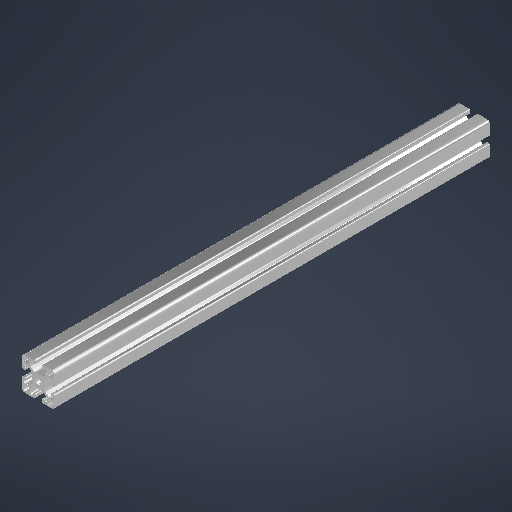
# Autodesk Inventor part: profileAluAvant2
Saved by Autodesk Inventor 2026.2 (Build 302298010, 298A)
## iProperties
Part Number: profileAluAvant2
Material: Générique
Document SubType Name: Modélisation
Designer: quent
Appearance: Par défaut
Author: quent
Autodesk Inventor part; units mm, degrees
ref_plane "Plan YZ" through (0, 0, 0) normal (1, 0, 0) x (0, 1, 0)
ref_plane "Plan XZ" through (0, 0, 0) normal (0, 1, 0) x (-1, 0, 0)
ref_plane "Plan XY" through (0, 0, 0) normal (0, 0, 1) x (1, 0, 0)
sketch "Esquisse1" plane through (0, 0, 0) normal (0, 0, 1) x (1, 0, 0)
  arc A0 (-0.1097, 10.4512) -> (1.0153, 9.3262) centre (1.0153, 10.4512) ccw
  line L0 (2.5153, 9.3262) -> (1.0153, 9.3262)
  arc A1 (2.5153, 9.3262) -> (3.2653, 10.0762) centre (2.5153, 10.0762) ccw
  line L1 (3.2653, 11.2012) -> (3.2653, 10.0762)
  arc A2 (3.2653, 11.2012) -> (2.8903, 11.5762) centre (2.8903, 11.2012) ccw
  line L2 (1.7653, 11.5762) -> (2.8903, 11.5762)
  arc A3 (1.3903, 11.9512) -> (1.7653, 11.5762) centre (1.7653, 11.9512) ccw
  arc A4 (3.2653, 13.8262) -> (1.3903, 11.9512) centre (3.2653, 11.9512) ccw
  line L3 (4.246, 13.8262) -> (3.2653, 13.8262)
  arc A5 (6.8976, 12.7279) -> (4.246, 13.8262) centre (4.246, 10.0762) ccw
  line L4 (7.9794, 11.6461) -> (6.8976, 12.7279)
  arc A6 (9.0778, 8.9944) -> (7.9794, 11.6461) centre (5.3278, 8.9944) ccw
  line L5 (9.0778, 3.658) -> (9.0778, 8.9944)
  arc A7 (7.9794, 1.0064) -> (9.0778, 3.658) centre (5.3278, 3.658) ccw
  line L6 (6.8976, -0.0754) -> (7.9794, 1.0064)
  arc A8 (4.246, -1.1738) -> (6.8976, -0.0754) centre (4.246, 2.5762) ccw
  line L7 (3.2653, -1.1738) -> (4.246, -1.1738)
  arc A9 (1.3903, 0.7012) -> (3.2653, -1.1738) centre (3.2653, 0.7012) ccw
  arc A10 (1.7653, 1.0762) -> (1.3903, 0.7012) centre (1.7653, 0.7012) ccw
  line L8 (2.8903, 1.0762) -> (1.7653, 1.0762)
  arc A11 (2.8903, 1.0762) -> (3.2653, 1.4512) centre (2.8903, 1.4512) ccw
  line L9 (3.2653, 2.5762) -> (3.2653, 1.4512)
  arc A12 (3.2653, 2.5762) -> (2.5153, 3.3262) centre (2.5153, 2.5762) ccw
  line L10 (1.0153, 3.3262) -> (2.5153, 3.3262)
  arc A13 (1.0153, 3.3262) -> (-0.1097, 2.2012) centre (1.0153, 2.2012) ccw
  line L11 (-0.1097, -5.6738) -> (-0.1097, 2.2012)
  arc A14 (-0.1097, -5.6738) -> (2.8903, -8.6738) centre (2.8903, -5.6738) ccw
  line L12 (10.7653, -8.6738) -> (2.8903, -8.6738)
  arc A15 (10.7653, -8.6738) -> (11.8903, -7.5488) centre (10.7653, -7.5488) ccw
  line L13 (11.8903, -6.0488) -> (11.8903, -7.5488)
  arc A16 (11.8903, -6.0488) -> (11.1403, -5.2988) centre (11.1403, -6.0488) ccw
  line L14 (10.0153, -5.2988) -> (11.1403, -5.2988)
  arc A17 (10.0153, -5.2988) -> (9.6403, -5.6738) centre (10.0153, -5.6738) ccw
  line L15 (9.6403, -6.7988) -> (9.6403, -5.6738)
  arc A18 (9.2653, -7.1738) -> (9.6403, -6.7988) centre (9.2653, -6.7988) ccw
  arc A19 (7.3903, -5.2988) -> (9.2653, -7.1738) centre (9.2653, -5.2988) ccw
  line L16 (7.3903, -4.3181) -> (7.3903, -5.2988)
  arc A20 (8.4886, -1.6664) -> (7.3903, -4.3181) centre (11.1403, -4.3181) ccw
  line L17 (9.5704, -0.5846) -> (8.4886, -1.6664)
  arc A21 (12.2221, 0.5137) -> (9.5704, -0.5846) centre (12.2221, -3.2363) ccw
  line L18 (17.5585, 0.5137) -> (12.2221, 0.5137)
  arc A22 (20.2101, -0.5846) -> (17.5585, 0.5137) centre (17.5585, -3.2363) ccw
  line L19 (21.2919, -1.6664) -> (20.2101, -0.5846)
  arc A23 (22.3903, -4.3181) -> (21.2919, -1.6664) centre (18.6403, -4.3181) ccw
  line L20 (22.3903, -5.2988) -> (22.3903, -4.3181)
  arc A24 (20.5153, -7.1738) -> (22.3903, -5.2988) centre (20.5153, -5.2988) ccw
  arc A25 (20.1403, -6.7988) -> (20.5153, -7.1738) centre (20.5153, -6.7988) ccw
  line L21 (20.1403, -5.6738) -> (20.1403, -6.7988)
  arc A26 (20.1403, -5.6738) -> (19.7653, -5.2988) centre (19.7653, -5.6738) ccw
  line L22 (18.6403, -5.2988) -> (19.7653, -5.2988)
  arc A27 (18.6403, -5.2988) -> (17.8903, -6.0488) centre (18.6403, -6.0488) ccw
  line L23 (17.8903, -7.5488) -> (17.8903, -6.0488)
  arc A28 (17.8903, -7.5488) -> (19.0153, -8.6738) centre (19.0153, -7.5488) ccw
  line L24 (26.8903, -8.6738) -> (19.0153, -8.6738)
  arc A29 (26.8903, -8.6738) -> (29.8903, -5.6738) centre (26.8903, -5.6738) ccw
  line L25 (29.8903, 2.2012) -> (29.8903, -5.6738)
  arc A30 (29.8903, 2.2012) -> (28.7653, 3.3262) centre (28.7653, 2.2012) ccw
  line L26 (27.2653, 3.3262) -> (28.7653, 3.3262)
  arc A31 (27.2653, 3.3262) -> (26.5153, 2.5762) centre (27.2653, 2.5762) ccw
  line L27 (26.5153, 1.4512) -> (26.5153, 2.5762)
  arc A32 (26.5153, 1.4512) -> (26.8903, 1.0762) centre (26.8903, 1.4512) ccw
  line L28 (28.0153, 1.0762) -> (26.8903, 1.0762)
  arc A33 (28.3903, 0.7012) -> (28.0153, 1.0762) centre (28.0153, 0.7012) ccw
  arc A34 (26.5153, -1.1738) -> (28.3903, 0.7012) centre (26.5153, 0.7012) ccw
  line L29 (25.5346, -1.1738) -> (26.5153, -1.1738)
  arc A35 (22.8829, -0.0754) -> (25.5346, -1.1738) centre (25.5346, 2.5762) ccw
  line L30 (21.8011, 1.0064) -> (22.8829, -0.0754)
  arc A36 (20.7028, 3.658) -> (21.8011, 1.0064) centre (24.4528, 3.658) ccw
  line L31 (20.7028, 8.9944) -> (20.7028, 3.658)
  arc A37 (21.8011, 11.6461) -> (20.7028, 8.9944) centre (24.4528, 8.9944) ccw
  line L32 (22.8829, 12.7279) -> (21.8011, 11.6461)
  arc A38 (25.5346, 13.8262) -> (22.8829, 12.7279) centre (25.5346, 10.0762) ccw
  line L33 (26.5153, 13.8262) -> (25.5346, 13.8262)
  arc A39 (28.3903, 11.9512) -> (26.5153, 13.8262) centre (26.5153, 11.9512) ccw
  arc A40 (28.0153, 11.5762) -> (28.3903, 11.9512) centre (28.0153, 11.9512) ccw
  line L34 (26.8903, 11.5762) -> (28.0153, 11.5762)
  arc A41 (26.8903, 11.5762) -> (26.5153, 11.2012) centre (26.8903, 11.2012) ccw
  line L35 (26.5153, 10.0762) -> (26.5153, 11.2012)
  arc A42 (26.5153, 10.0762) -> (27.2653, 9.3262) centre (27.2653, 10.0762) ccw
  line L36 (28.7653, 9.3262) -> (27.2653, 9.3262)
  arc A43 (28.7653, 9.3262) -> (29.8903, 10.4512) centre (28.7653, 10.4512) ccw
  line L37 (29.8903, 18.3262) -> (29.8903, 10.4512)
  arc A44 (29.8903, 18.3262) -> (26.8903, 21.3262) centre (26.8903, 18.3262) ccw
  line L38 (19.0153, 21.3262) -> (26.8903, 21.3262)
  arc A45 (19.0153, 21.3262) -> (17.8903, 20.2012) centre (19.0153, 20.2012) ccw
  line L39 (17.8903, 18.7012) -> (17.8903, 20.2012)
  arc A46 (17.8903, 18.7012) -> (18.6403, 17.9512) centre (18.6403, 18.7012) ccw
  line L40 (19.7653, 17.9512) -> (18.6403, 17.9512)
  arc A47 (19.7653, 17.9512) -> (20.1403, 18.3262) centre (19.7653, 18.3262) ccw
  line L41 (20.1403, 19.4512) -> (20.1403, 18.3262)
  arc A48 (20.5153, 19.8262) -> (20.1403, 19.4512) centre (20.5153, 19.4512) ccw
  arc A49 (22.3903, 17.9512) -> (20.5153, 19.8262) centre (20.5153, 17.9512) ccw
  line L42 (22.3903, 16.9705) -> (22.3903, 17.9512)
  arc A50 (21.2919, 14.3189) -> (22.3903, 16.9705) centre (18.6403, 16.9705) ccw
  line L43 (20.2101, 13.2371) -> (21.2919, 14.3189)
  arc A51 (17.5585, 12.1387) -> (20.2101, 13.2371) centre (17.5585, 15.8887) ccw
  line L44 (12.2221, 12.1387) -> (17.5585, 12.1387)
  arc A52 (9.5704, 13.2371) -> (12.2221, 12.1387) centre (12.2221, 15.8887) ccw
  line L45 (8.4886, 14.3189) -> (9.5704, 13.2371)
  arc A53 (7.3903, 16.9705) -> (8.4886, 14.3189) centre (11.1403, 16.9705) ccw
  line L46 (7.3903, 17.9512) -> (7.3903, 16.9705)
  arc A54 (9.2653, 19.8262) -> (7.3903, 17.9512) centre (9.2653, 17.9512) ccw
  arc A55 (9.6403, 19.4512) -> (9.2653, 19.8262) centre (9.2653, 19.4512) ccw
  line L47 (9.6403, 18.3262) -> (9.6403, 19.4512)
  arc A56 (9.6403, 18.3262) -> (10.0153, 17.9512) centre (10.0153, 18.3262) ccw
  line L48 (11.1403, 17.9512) -> (10.0153, 17.9512)
  arc A57 (11.1403, 17.9512) -> (11.8903, 18.7012) centre (11.1403, 18.7012) ccw
  line L49 (11.8903, 20.2012) -> (11.8903, 18.7012)
  arc A58 (11.8903, 20.2012) -> (10.7653, 21.3262) centre (10.7653, 20.2012) ccw
  line L50 (2.8903, 21.3262) -> (10.7653, 21.3262)
  arc A59 (2.8903, 21.3262) -> (-0.1097, 18.3262) centre (2.8903, 18.3262) ccw
  line L51 (-0.1097, 10.4512) -> (-0.1097, 18.3262)
  line L52 (23.7403, -6.9488) -> (23.7403, -2.8988)
  arc A60 (24.1153, -2.5238) -> (23.7403, -2.8988) centre (24.1153, -2.8988) ccw
  line L53 (24.1153, -2.5238) -> (28.1653, -2.5238)
  arc A61 (28.5403, -2.8988) -> (28.1653, -2.5238) centre (28.1653, -2.8988) ccw
  line L54 (28.5403, -2.8988) -> (28.5403, -5.6738)
  arc A62 (26.8903, -7.3238) -> (28.5403, -5.6738) centre (26.8903, -5.6738) ccw
  line L55 (26.8903, -7.3238) -> (24.1153, -7.3238)
  arc A63 (23.7403, -6.9488) -> (24.1153, -7.3238) centre (24.1153, -6.9488) ccw
  line L56 (1.6153, -2.5238) -> (5.6653, -2.5238)
  arc A64 (6.0403, -2.8988) -> (5.6653, -2.5238) centre (5.6653, -2.8988) ccw
  line L57 (6.0403, -2.8988) -> (6.0403, -6.9488)
  arc A65 (5.6653, -7.3238) -> (6.0403, -6.9488) centre (5.6653, -6.9488) ccw
  line L58 (5.6653, -7.3238) -> (2.8903, -7.3238)
  arc A66 (1.2403, -5.6738) -> (2.8903, -7.3238) centre (2.8903, -5.6738) ccw
  line L59 (1.2403, -5.6738) -> (1.2403, -2.8988)
  arc A67 (1.6153, -2.5238) -> (1.2403, -2.8988) centre (1.6153, -2.8988) ccw
  line L60 (6.0403, 19.6012) -> (6.0403, 15.5512)
  arc A68 (5.6653, 15.1762) -> (6.0403, 15.5512) centre (5.6653, 15.5512) ccw
  line L61 (5.6653, 15.1762) -> (1.6153, 15.1762)
  arc A69 (1.2403, 15.5512) -> (1.6153, 15.1762) centre (1.6153, 15.5512) ccw
  line L62 (1.2403, 15.5512) -> (1.2403, 18.3262)
  arc A70 (2.8903, 19.9762) -> (1.2403, 18.3262) centre (2.8903, 18.3262) ccw
  line L63 (2.8903, 19.9762) -> (5.6653, 19.9762)
  arc A71 (6.0403, 19.6012) -> (5.6653, 19.9762) centre (5.6653, 19.6012) ccw
  line L64 (28.1653, 15.1762) -> (24.1153, 15.1762)
  arc A72 (23.7403, 15.5512) -> (24.1153, 15.1762) centre (24.1153, 15.5512) ccw
  line L65 (23.7403, 15.5512) -> (23.7403, 19.6012)
  arc A73 (24.1153, 19.9762) -> (23.7403, 19.6012) centre (24.1153, 19.6012) ccw
  line L66 (24.1153, 19.9762) -> (26.8903, 19.9762)
  arc A74 (28.5403, 18.3262) -> (26.8903, 19.9762) centre (26.8903, 18.3262) ccw
  line L67 (28.5403, 18.3262) -> (28.5403, 15.5512)
  arc A75 (28.1653, 15.1762) -> (28.5403, 15.5512) centre (28.1653, 15.5512) ccw
  circle A76 centre (14.8903, 6.3262) radius 2.55
  point P0 (0, 0)
  point P1 (11.3248, 5.3075)
  point P2 (11.9403, 10.0762)
  constraints: 152 point on circle, 136 end point, 77 centre point
extrude "Extrusion1" add sketch "Esquisse1" along normal blind 394.7
